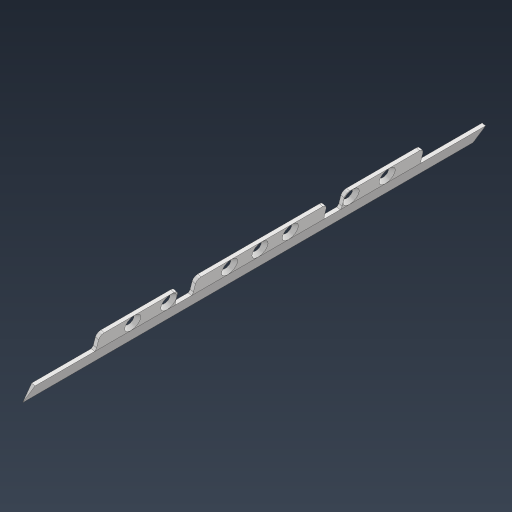
# Autodesk Inventor part: blade-uphold
Saved by Autodesk Inventor 2023 (Build 270158000, 158)
## iProperties
Created: 2025-10-16
Part Number: blade-uphold
Material: Generic
Document SubType Name: Modeling
Designer: szymo
Density: 1 g/cm^3
Appearance: Default
Author: szymo
Autodesk Inventor part; units mm, degrees
ref_plane "YZ Plane" through (0, 0, 0) normal (1, 0, 0) x (0, 1, 0)
ref_plane "XZ Plane" through (0, 0, 0) normal (0, 1, 0) x (-1, 0, 0)
sketch "Sketch1" plane through (0, 0, 0) normal (0, 0, 1) x (1, 0, 0)
  line L0 (1.904, 4.8961) -> (-3.8986, -12.143) projected
  line L1 (-3.8986, -12.143) -> (-3.7093, -12.2075) projected
  line L2 (2.0933, 4.8316) -> (-3.7093, -12.2075) projected
  line L3 (1.904, 4.8961) -> (2.0933, 4.8316) projected
  line L4 (-2.2093, -5.6314) -> (-0.2093, 1.7925) projected
  line L5 (-1.736, -5.7925) -> (-2.2093, -5.6314) projected
  line L6 (2.2093, 5.7925) -> (-1.736, -5.7925) projected
  line L7 (-0.2093, 5.7925) -> (2.2093, 5.7925) projected
  line L8 (-0.2093, 1.7925) -> (-0.2093, 5.7925) projected
  line L9 (4.4659, 12.4188) -> (2.2093, 5.7925) projected
  line L10 (2.2093, 14.9971) -> (4.4659, 12.4188) projected
  line L11 (2.2093, 5.7925) -> (2.2093, 14.9971) projected
  line L12 (-0.9019, -3.9638) -> (4.6128, 5.222)
  line L13 (4.6128, 5.222) -> (6.3106, 12.013)
  line L14 (6.3106, 12.013) -> (4.8659, 12.4188)
  line L15 (4.8659, 12.4188) -> (3.2093, 5.7925)
  line L16 (3.2093, 5.7925) -> (-0.9019, -3.9638)
  line L17 (4.8659, 12.4188) -> (4.4659, 12.4188) construction
  line L18 (2.2093, 5.7925) -> (3.2093, 5.7925) construction
  line L19 (4.0065, 8.9813) -> (5.4617, 8.6175)
  line L20 (2.1389, 7.137) -> (3.5896, 11.3968) projected
  point P0 (0, 0)
  dimension "d0" = 0.4
  dimension "d1" = 1
  dimension "d2" = 2
  dimension "d3" = 1.5
  dimension "d4" = 2.2422
  dimension "d5" = 2.2422
  dimension "d6" = 3.5
  dimension "d7" = 3.5
  constraints: 16 end point, 2 horizontal, 2 perpendicular, 2 point on line, 1 midpoint
  measures "d0" distance of L14.end L9.start
  measures "d1" distance of L6.start L15.end
  measures "d2" distance from line of L5 L12.start
  measures "d3" distance of L19.start L19.end
  measures "d4" distance from line of L19 L20.end
  measures "d5" distance from line of L19 L20.start
  measures "d6" distance from line of L19 L12.end
  measures "d7" distance from line of L13.end L19
ref_plane "Work Plane1" through (-2.2093, -5.7925, -200) normal (0, 0, -1) x (0, 1, 0)
extrude "Extrusion1" add sketch "Sketch1" against normal up to surface (200 mm away) contours L16 L15 L19 L13 L12 | L19 L15 L14 L13
sketch "Sketch2" plane through (6.3106, 12.013, 0) normal (0.9701425, -0.2425356, 0) x (0, 0, -1)
  line L0 (200, -7) -> (200, 0) projected
  line L1 (0, 0) -> (200, 0) projected
  line L2 (0, -7) -> (0, 0) projected
  line L3 (0, -7) -> (200, -7) projected
  ellipse E0 centre (139.5, -3.2921) end of major axis (137.5, -3.2921) minor radius 1.9931 projected
  ellipse E1 centre (155.5, -3.2921) end of major axis (153.5, -3.2921) minor radius 1.9931 projected
  ellipse E2 centre (112.5, -3.2921) end of major axis (110.5, -3.2921) minor radius 1.9931 projected
  ellipse E3 centre (99, -3.2921) end of major axis (97, -3.2921) minor radius 1.9931 projected
  ellipse E4 centre (85.5, -3.2921) end of major axis (83.5, -3.2921) minor radius 1.9931 projected
  ellipse E5 centre (58.5, -3.2921) end of major axis (56.5, -3.2921) minor radius 1.9931 projected
  ellipse E6 centre (42.5, -3.2921) end of major axis (40.5, -3.2921) minor radius 1.9931 projected
  line L4 (42.5, 0) -> (42.5, -7) construction
  line L5 (58.5, 0) -> (58.5, -7) construction
  line L6 (85.5, 0) -> (85.5, -7) construction
  line L7 (99, -7) -> (99, 0) construction
  line L8 (112.5, 0) -> (112.5, -7) construction
  line L9 (139.5, 0) -> (139.5, -7) construction
  line L10 (155.5, -7) -> (155.5, 0) construction
  line L11 (33.0563, -3.5) -> (172.1416, -3.5) construction
  point P0 (0, -13.1849)
  point P1 (42.5, -3.5)
  point P2 (58.5, -3.5)
  point P3 (85.5, -3.5)
  point P4 (99, -3.5)
  point P5 (112.5, -3.5)
  point P6 (155.5, -3.5)
  point P7 (139.5, -3.5)
  dimension "d11" = 3.5
  constraints: 14 end point, 9 vertical, 7 midpoint, 7 point on line, 33 other
hole "Hole1" at (5.4617, 8.6175, -42.5) at (5.4617, 8.6175, -58.5) at (5.4617, 8.6175, -85.5) at (5.4617, 8.6175, -99) at (5.4617, 8.6175, -112.5) at (5.4617, 8.6175, -155.5) at (5.4617, 8.6175, -139.5) direction (-0.9701425, 0.2425356, 0) diameter 3.6 depth 3 countersink diameter 7 countersink angle 90 clearance for "Countersunk Flat Head Screw ISO 2009/7046" size "M3" standard "ISO"
fillet "Fillet1" radius 10 1 edges at (3.2093, 5.7925, -100)
sketch "Sketch4" plane through (6.3106, 12.013, 0) normal (0.9701425, -0.2425356, 0) x (0, 0, -1)
  line L0 (0, 0.0433) -> (200, 0.0433) projected
  line L1 (0, -7) -> (42.5, -7) projected
  line L2 (42.5, -7) -> (58.5, -7) projected
  line L3 (58.5, -7) -> (85.5, -7) projected
  line L4 (85.5, -7) -> (99, -7) projected
  line L5 (99, -7) -> (112.5, -7) projected
  line L6 (112.5, -7) -> (139.5, -7) projected
  line L7 (139.5, -7) -> (155.5, -7) projected
  line L8 (155.5, -7) -> (200, -7) projected
  line L9 (200, -7) -> (200, 0) projected
  line L10 (0, -7) -> (0, 0) projected
  line L11 (0, 0) -> (0, 0.0433) projected
  line L12 (200, 0) -> (200, 0.0433) projected
  ellipse E0 centre (169, 1.1152) end of major axis (167, 1.1152) minor radius 1.9403 (171, 1.1152) -> (169, 3.0555) ccw projected
  line L13 (171, 1.1152) -> (171, -5.6758) projected
  ellipse E1 centre (173, -5.6758) end of major axis (171, -5.6758) minor radius 1.9403 (171, -5.6758) -> (173, -7.616) ccw projected
  line L14 (173, -7.616) -> (200, -7.616) projected
  line L15 (200, -7.616) -> (200, -11.4966) projected
  line L16 (0, -11.4966) -> (200, -11.4966) projected
  line L17 (0, -11.4966) -> (0, -7.616) projected
  line L18 (0, -7.616) -> (25, -7.616) projected
  ellipse E2 centre (25, -5.6758) end of major axis (23, -5.6758) minor radius 1.9403 (25, -7.616) -> (27, -5.6758) ccw projected
  line L19 (27, -5.6758) -> (27, 1.1152) projected
  ellipse E3 centre (29, 1.1152) end of major axis (27, 1.1152) minor radius 1.9403 (29, 3.0555) -> (27, 1.1152) ccw projected
  line L20 (60, 3.0555) -> (29, 3.0555) projected
  ellipse E4 centre (60, 1.1152) end of major axis (58, 1.1152) minor radius 1.9403 (62, 1.1152) -> (60, 3.0555) ccw projected
  line L21 (62, -5.6758) -> (62, 1.1152) projected
  ellipse E5 centre (64, -5.6758) end of major axis (62, -5.6758) minor radius 1.9403 (62, -5.6758) -> (64, -7.616) ccw projected
  line L22 (64, -7.616) -> (68, -7.616) projected
  ellipse E6 centre (68, -5.6758) end of major axis (66, -5.6758) minor radius 1.9403 (68, -7.616) -> (70, -5.6758) ccw projected
  line L23 (70, -5.6758) -> (70, 1.1152) projected
  ellipse E7 centre (72, 1.1152) end of major axis (70, 1.1152) minor radius 1.9403 (72, 3.0555) -> (70, 1.1152) ccw projected
  line L24 (126, 3.0555) -> (72, 3.0555) projected
  ellipse E8 centre (126, 1.1152) end of major axis (124, 1.1152) minor radius 1.9403 (128, 1.1152) -> (126, 3.0555) ccw projected
  line L25 (128, 1.1152) -> (128, -5.6758) projected
  ellipse E9 centre (130, -5.6758) end of major axis (128, -5.6758) minor radius 1.9403 (128, -5.6758) -> (130, -7.616) ccw projected
  line L26 (130, -7.616) -> (134, -7.616) projected
  ellipse E10 centre (134, -5.6758) end of major axis (132, -5.6758) minor radius 1.9403 (134, -7.616) -> (136, -5.6758) ccw projected
  line L27 (136, 1.1152) -> (136, -5.6758) projected
  ellipse E11 centre (138, 1.1152) end of major axis (136, 1.1152) minor radius 1.9403 (138, 3.0555) -> (136, 1.1152) ccw projected
  line L28 (169, 3.0555) -> (138, 3.0555) projected
  ellipse E12 centre (77.5, -3.7355) end of major axis (75.5, -3.7355) minor radius 1.9403 projected
  ellipse E13 centre (163.5, -3.7355) end of major axis (161.5, -3.7355) minor radius 1.9403 projected
  ellipse E14 centre (120.5, -3.7355) end of major axis (118.5, -3.7355) minor radius 1.9403 projected
  ellipse E15 centre (34.5, -3.7355) end of major axis (32.5, -3.7355) minor radius 1.9403 projected
  point P0 (0, -13.1849)
  point P1 (171, 0.0433)
  point P2 (171.5382, -7)
  point P3 (136, 0.0433)
  point P4 (128, 0.0433)
  point P5 (128.5382, -7)
  point P6 (135.4618, -7)
  point P7 (70, 0.0433)
  point P8 (62, 0.0433)
  point P9 (62.5382, -7)
  point P10 (69.4618, -7)
  point P11 (26.4618, -7)
  point P12 (27, 0.0433)
  constraints: 16 other
extrude "Extrusion3" cut sketch "Sketch4" against normal blind 10 contours L0 L19 E2 L1 L10 L11 | L0 L23 E6 L3 E5 L21 | L0 L27 E10 L6 E9 L25 | L0 L12 L9 L8 E1 L13
fillet "Fillet2" radius 2 6 edges at (5.5882, 12.2159, -27) (5.5882, 12.2159, -62) (5.5882, 12.2159, -70) (5.5882, 12.2159, -128) (5.5882, 12.2159, -136) (5.5882, 12.2159, -171)
equation "\"d4\" = d5"
equation "\"d6\" = d7"
body "Solid1"
